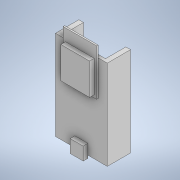
# Autodesk Inventor part: ESP32-DevKitC
Saved by Autodesk Inventor 2022 (Build 260153000, 153)
## iProperties
Created: 2024-06-27
Part Number: ESP32-DevKitC
Material: 一般
Document SubType Name: Modeling
Designer: yamashita1
Density: 1 g/cm^3
Appearance: 既定
Author: yamashita1
Autodesk Inventor part; units mm, degrees
ref_plane "YZ Plane" through (0, 0, 0) normal (1, 0, 0) x (0, 1, 0)
ref_plane "XZ Plane" through (0, 0, 0) normal (0, 1, 0) x (-1, 0, 0)
ref_plane "XY Plane" through (0, 0, 0) normal (0, 0, 1) x (1, 0, 0)
sketch "スケッチ1" plane through (0, 0, 0) normal (0, 0, 1) x (1, 0, 0)
  line L0 (-13.97, 24.13) -> (13.97, 24.13)
  line L1 (13.97, 24.13) -> (13.97, -24.13)
  line L2 (13.97, -24.13) -> (-13.97, -24.13)
  line L3 (-13.97, -24.13) -> (-13.97, 24.13)
  point P0 (0, 0)
  point P1 (-13.97, 0)
  point P2 (0, -24.13)
  dimension "d0" = 27.94
  dimension "d1" = 48.26
  constraints: 8 end point, 2 midpoint, 2 parallel, 1 horizontal, 1 horizontal alignment, 1 perpendicular, 1 vertical alignment
  measures "d0" distance of L1.end L2.end
  measures "d1" distance of L0.end L1.end
extrude "押し出し1" add sketch "スケッチ1" along normal blind 1.6
sketch "スケッチ2" plane through (0, 0, 0) normal (0, 0, -1) x (-1, 0, 0)
  line L0 (0, 28.1996) -> (0, -28.1996) construction
  line L1 (-12.7, -28.1996) -> (-12.7, 28.1996) construction
  line L2 (12.7, 28.1996) -> (12.7, -28.1996) construction
  line L3 (-11.43, 24.13) -> (-13.97, 24.13)
  line L4 (-13.97, 24.13) -> (-13.97, -24.13)
  line L5 (-13.97, -24.13) -> (-11.43, -24.13)
  line L6 (-11.43, -24.13) -> (-11.43, 24.13)
  line L7 (11.43, 24.13) -> (13.97, 24.13)
  line L8 (13.97, 24.13) -> (13.97, -24.13)
  line L9 (13.97, -24.13) -> (11.43, -24.13)
  line L10 (11.43, -24.13) -> (11.43, 24.13)
  line L11 (-13.97, -24.13) -> (-13.97, 24.13) projected
  line L12 (-13.97, 24.13) -> (13.97, 24.13) projected
  line L13 (13.97, 24.13) -> (13.97, -24.13) projected
  line L14 (13.97, -24.13) -> (-13.97, -24.13) projected
  point P0 (0, 0)
  point P1 (0, 0)
  point P2 (-12.7, 24.13)
  point P3 (12.7, 24.13)
  dimension "d4" = 25.4
  dimension "d5" = 2.54
  constraints: 22 end point, 6 collinear, 4 parallel, 3 horizontal alignment, 3 midpoint, 2 horizontal, 2 perpendicular, 2 point on line, 1 coincident, 1 vertical, 1 other
  measures "d4" distance of L2.start L1.end
  measures "d5" distance of L4.end L5.end
extrude "押し出し2" add sketch "スケッチ2" along normal blind 11 contours L6 L5 L4 L3 | L7 L8 L9 L10
sketch "スケッチ3" plane through (0, 0, 1.6) normal (0, 0, 1) x (1, 0, 0)
  line L0 (-9, 30.13) -> (9, 30.13)
  line L1 (9, 30.13) -> (9, 5.13)
  line L2 (9, 5.13) -> (-9, 5.13)
  line L3 (-9, 5.13) -> (-9, 30.13)
  line L4 (13.97, 24.13) -> (-13.97, 24.13) projected
  point P0 (0, 0)
  point P1 (0, 5.13)
  dimension "d8" = 18
  dimension "d9" = 25
  dimension "d10" = 6
  constraints: 8 end point, 2 parallel, 1 horizontal, 1 midpoint, 1 perpendicular, 1 vertical alignment
  measures "d8" distance of L1.end L2.end
  measures "d9" distance of L0.end L1.end
  measures "d10" distance between parallel lines of L4 L0
extrude "押し出し3" add sketch "スケッチ3" along normal blind 0.8
sketch "スケッチ4" plane through (0, 0, 2.4) normal (0, 0, 1) x (1, 0, 0)
  line L0 (-7.75, 23.63) -> (7.75, 23.63)
  line L1 (7.75, 23.63) -> (7.75, 6.63)
  line L2 (7.75, 6.63) -> (-7.75, 6.63)
  line L3 (-7.75, 6.63) -> (-7.75, 23.63)
  line L4 (-9, 5.13) -> (9, 5.13) projected
  point P0 (0, 0)
  point P1 (0, 6.63)
  dimension "d13" = 15.5
  dimension "d14" = 17
  dimension "d15" = 1.5
  constraints: 8 end point, 2 parallel, 1 horizontal, 1 midpoint, 1 perpendicular, 1 vertical alignment
  measures "d13" distance of L1.end L2.end
  measures "d14" distance of L0.end L1.end
  measures "d15" distance between parallel lines of L4 L2
extrude "押し出し4" add sketch "スケッチ4" along normal blind 2.5
sketch "スケッチ5" plane through (0, 0, 1.6) normal (0, 0, 1) x (1, 0, 0)
  line L0 (-3.5, -18.63) -> (3.5, -18.63)
  line L1 (3.5, -18.63) -> (3.5, -25.63)
  line L2 (3.5, -25.63) -> (-3.5, -25.63)
  line L3 (-3.5, -25.63) -> (-3.5, -18.63)
  line L4 (-13.97, -24.13) -> (13.97, -24.13) projected
  point P0 (0, 0)
  point P1 (0, -18.63)
  dimension "d18" = 7
  dimension "d19" = 7
  dimension "d20" = 1.5
  constraints: 8 end point, 2 parallel, 1 horizontal, 1 midpoint, 1 perpendicular, 1 vertical alignment
  measures "d18" distance of L1.end L2.end
  measures "d19" distance of L0.end L1.end
  measures "d20" distance between parallel lines of L2 L4
extrude "押し出し5" add sketch "スケッチ5" along normal blind 2.5
